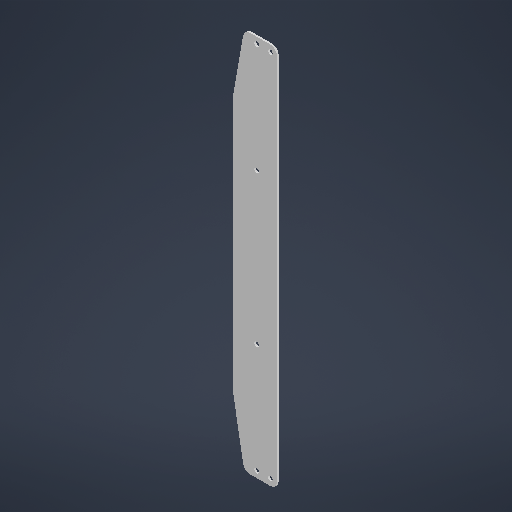
# Autodesk Inventor part: sidePlates
Saved by Autodesk Inventor 2025.1 (Build 291241000, 241)
## iProperties
Created: 2025-01-10
Part Number: sidePlates
Material: Generic
Document SubType Name: Modeling
Designer: Jahan
Density: 1 g/cm^3
Appearance: Default
Author: Jahan
Autodesk Inventor part; units mm, degrees
ref_plane "YZ Plane" through (0, 0, 0) normal (1, 0, 0) x (0, 1, 0)
ref_plane "XZ Plane" through (0, 0, 0) normal (0, 1, 0) x (-1, 0, 0)
ref_plane "XY Plane" through (0, 0, 0) normal (0, 0, 1) x (1, 0, 0)
sketch "Sketch1" plane through (0, 0, 0) normal (0, 0, 1) x (1, 0, 0)
  circle A0 centre (12.8898, 175.1935) radius 2.1844
  circle A1 centre (12.8898, -167.7065) radius 2.1844
  circle A2 centre (0.1898, 73.5935) radius 2.1844
  circle A3 centre (0.1898, -66.1065) radius 2.1844
  circle A4 centre (0.1898, 175.1935) radius 2.1844
  circle A5 centre (0.1898, -167.7065) radius 2.1844
  arc A6 (18.9223, 175.1935) -> (12.8898, 181.226) centre (12.8898, 175.1935) ccw
  arc A7 (12.8898, -173.739) -> (18.9223, -167.7065) centre (12.8898, -167.7065) ccw
  arc A8 (18.9223, 175.1935) -> (12.8898, 181.226) centre (12.8898, 175.1935) ccw
  line L0 (18.9223, 175.1935) -> (18.9223, -167.7065)
  line L1 (12.8898, 181.226) -> (-6.1602, 181.226)
  line L2 (-6.1602, 181.226) -> (-6.1602, 181.226)
  arc A9 (-6.1602, 181.226) -> (-12.4137, 175.9786) centre (-6.1602, 174.876) ccw
  line L3 (-6.1602, 181.226) -> (-6.1602, 174.876) construction
  line L4 (-12.4137, 175.9786) -> (-6.1602, 174.876) construction
  line L5 (-12.4137, 175.9786) -> (-21.235, 125.9504)
  arc A10 (-21.235, 125.9504) -> (-21.428, 123.7451) centre (-8.728, 123.7451) ccw
  line L6 (-21.235, 125.9504) -> (-8.728, 123.7451) construction
  line L7 (-21.428, 123.7451) -> (-8.728, 123.7451) construction
  line L8 (18.9223, 3.7435) -> (0.1898, 3.7435)
  line L9 (-21.428, -116.2581) -> (-8.728, -116.2581) construction
  arc A11 (-21.428, -116.2581) -> (-21.235, -118.4635) centre (-8.728, -116.2581) ccw
  line L10 (-21.235, -118.4635) -> (-8.728, -116.2581) construction
  line L11 (-12.4137, -168.4917) -> (-21.235, -118.4635)
  line L12 (-12.4137, -168.4917) -> (-6.1602, -167.389) construction
  arc A12 (-12.4137, -168.4917) -> (-6.1602, -173.739) centre (-6.1602, -167.389) ccw
  line L13 (-6.1602, -173.739) -> (-6.1602, -173.739)
  line L14 (12.8898, -173.739) -> (-6.1602, -173.739)
  line L15 (-6.1602, -173.739) -> (-6.1602, -167.389) construction
  line L16 (-21.428, -116.2581) -> (-21.428, 123.7451)
  point P0 (0, 0)
  point P1 (12.8898, -167.7065)
  point P2 (0.1898, -167.7065)
  point P3 (12.8898, -167.7065)
  point P4 (12.8898, -167.7065)
  point P5 (-6.1602, -173.739)
  dimension "d1" = 6.35
  dimension "d2" = 80
  dimension "d3" = 50.8
  dimension "d4" = 12.7
  dimension "d5" = 10
  dimension "d15" = 19.05
  constraints: 34 end point, 14 point on circle, 13 centre point, 11 symmetric about line, 3 coincident, 3 tangent, 2 horizontal, 2 vertical, 1 midpoint, 2 other
  measures "d1" radius of A9
  measures "d2" angle of L3 L4
  measures "d3" distance of L5.start L6.start
  measures "d4" radius of A10
  measures "d5" angle of L6 L7
  measures "d15" distance of L1.start L2.start
extrude "Extrusion2" add sketch "Sketch1" along normal blind 1.5875
body "Solid2"
